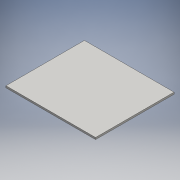
# Autodesk Inventor part: Bucket - door 2
Saved by Autodesk Inventor 2016 (Build 200138000, 138)
## iProperties
Created: 2016-01-14
Part Number: Bucket - door 2
Material: Generic
Document SubType Name: Modeling
Designer: TimB
Density: 1 g/cm^3
Appearance: Default
Author: TimB
Autodesk Inventor part; units mm, degrees
ref_plane "YZ Plane" through (0, 0, 0) normal (1, 0, 0) x (0, 1, 0)
ref_plane "XZ Plane" through (0, 0, 0) normal (0, 1, 0) x (-1, 0, 0)
ref_plane "XY Plane" through (0, 0, 0) normal (0, 0, 1) x (1, 0, 0)
sketch "Sketch1" plane through (0, 0, 0) normal (0, 0, 1) x (1, 0, 0)
  line L0 (72.5, 63.5) -> (-72.5, 63.5)
  line L1 (-72.5, 63.5) -> (-72.5, -63.5)
  line L2 (-72.5, -63.5) -> (72.5, -63.5)
  line L3 (72.5, -63.5) -> (72.5, 63.5)
  line L4 (72.5, 63.5) -> (-72.5, -63.5) construction
  line L5 (-72.5, 63.5) -> (72.5, -63.5) construction
  circle A0 centre (33.08, -58.41) radius 2.85 projected
  line L6 (42.7414, -68.16) -> (3.4186, -68.16) projected
  line L7 (-72.5, -38.1) -> (-68.69, -38.1) projected
  line L8 (-3.32, -64.81) -> (-3.32, -66.86) projected
  point P0 (0, 0)
  dimension "d0" = 145
  dimension "d1" = 127
  constraints: 12 end point, 2 midpoint, 2 parallel, 1 horizontal, 1 perpendicular
  measures "d0" distance of L2.end L1.end
  measures "d1" distance of L1.end L0.end
extrude "Extrusion1" add sketch "Sketch1" along normal blind 3 contours L3 L2 L1 L0 | A0
body "Solid1"
